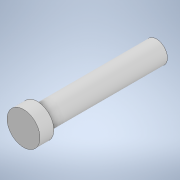
# Autodesk Inventor part: pin-1
Saved by Autodesk Inventor 2020 (Build 240168000, 168)
## iProperties
Created: 2021-05-09
Part Number: pin-1
Material: Generic
Document SubType Name: Modeling
Designer: Hengameh
Density: 1 g/cm^3
Appearance: Default
Author: Hengameh
Autodesk Inventor part; units mm, degrees
ref_plane "YZ Plane" through (0, 0, 0) normal (1, 0, 0) x (0, 1, 0)
ref_plane "XZ Plane" through (0, 0, 0) normal (0, 1, 0) x (-1, 0, 0)
ref_plane "XY Plane" through (0, 0, 0) normal (0, 0, 1) x (1, 0, 0)
sketch "Sketch1" plane through (0, 0, 0) normal (0, 0, 1) x (1, 0, 0)
  circle A0 centre (0, 0) radius 4.15
  dimension "PIN_DIA" = 8.3
  constraints: 1 centre point, 1 coincident
  measures "PIN_DIA" diameter of A0
extrude "Extrusion1" add sketch "Sketch1" along normal mid plane 45
sketch "Sketch2" plane through (0, 0, 22.5) normal (0, 0, 1) x (1, 0, 0)
  circle A0 centre (0, 0) radius 6.225
  dimension "PIN_HEAD_DIA" = 12.45
  constraints: 1 centre point, 1 coincident
  measures "PIN_HEAD_DIA" diameter of A0
extrude "Extrusion2" add sketch "Sketch2" along normal blind 5.229
equation "\"PIN_HEAD_DIA\" = 1.5 * PIN_DIA"
equation "\"PIN_HEAD_H\" = 0.42 * PIN_HEAD_DIA"
body "Solid1"
